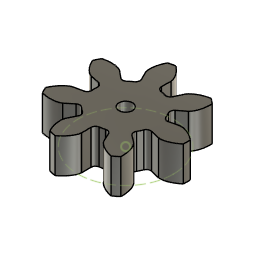
Motor Gear v04 (Autodesk Fusion 360 design; units mm, degrees)
description: Spur Gear; Module: 5.0; Num Teeth: 7; Pressure Angle: 20.0; Backlash: 0.00 mm
Autodesk Fusion 360 part; units mm, degrees
sketch "Sketch1" plane through (0, 0, 0) normal (0, 0, 1) x (1, 0, 0) in component "Spur Gear (7 teeth)"
  circle A0 centre (0, 0) radius 11.4492
  circle A1 centre (0, 0) radius 2.5
extrude "Extrude1" add sketch "Sketch1" along normal blind 12.7 in component "Spur Gear (7 teeth)"
sketch "Sketch2" plane through (0, 0, 0) normal (0, 0, 1) x (1, 0, 0) in component "Spur Gear (7 teeth)"
  spline S0 degree 5 poles (15.976, -3.8978) (15.9941, -3.9022) (16.0303, -3.9103) (16.085, -3.9201) (16.1585, -3.9291) (16.2513, -3.9345) (16.3447, -3.936) (16.4386, -3.9351) (16.5326, -3.9328) (16.6268, -3.9296) (16.7211, -3.9253) (16.8156, -3.9196) (16.9102, -3.912) (17.0051, -3.9022) (17.1001, -3.8904) (17.1953, -3.8767) (17.2906, -3.8614) (17.386, -3.8448) (17.4814, -3.827) (17.5768, -3.808) (17.6722, -3.7879) (17.7676, -3.7664) (17.8631, -3.7436) (17.9586, -3.7194) (18.054, -3.694) (18.1494, -3.6672) (18.2448, -3.6393) (18.3402, -3.6102) (18.4355, -3.58) (18.5307, -3.5487) (18.6259, -3.5163) (18.7209, -3.4828) (18.8159, -3.4482) (18.9108, -3.4124) (19.0056, -3.3756) (19.1003, -3.3378) (19.1948, -3.2988) (19.2893, -3.2589) (19.3835, -3.2179) (19.4777, -3.1759) (19.5717, -3.133) (19.6655, -3.089) (19.7592, -3.044) (19.8527, -2.9981) (19.946, -2.9512) (20.0392, -2.9033) (20.1321, -2.8545) (20.2249, -2.8047) (20.3175, -2.7541) (20.4098, -2.7024) (20.502, -2.6499) (20.5939, -2.5964) (20.6856, -2.5421) (20.7771, -2.4868) (20.8683, -2.4307) (20.9593, -2.3737) (21.05, -2.3157) (21.1405, -2.257) (21.2307, -2.1973) (21.3207, -2.1368) (21.4104, -2.0754) (21.4998, -2.0132) (21.589, -1.9502) (21.6778, -1.8863) (21.7664, -1.8215) (21.8547, -1.756) (21.9427, -1.6896) (22.0303, -1.6224) (22.1177, -1.5544) (22.2047, -1.4857) (22.2915, -1.4161) (22.3606, -1.3598) (22.4123, -1.3172) (22.4467, -1.2886) (22.4639, -1.2743) knots 0 0 0 0 0 0 0.01428571 0.02857143 0.04285714 0.05714286 0.07142857 0.08571429 0.1 0.11428571 0.12857143 0.14285714 0.15714286 0.17142857 0.18571429 0.2 0.21428571 0.22857143 0.24285714 0.25714286 0.27142857 0.28571429 0.3 0.31428571 0.32857143 0.34285714 0.35714286 0.37142857 0.38571429 0.4 0.41428571 0.42857143 0.44285714 0.45714286 0.47142857 0.48571429 0.5 0.51428571 0.52857143 0.54285714 0.55714286 0.57142857 0.58571429 0.6 0.61428571 0.62857143 0.64285714 0.65714286 0.67142857 0.68571429 0.7 0.71428571 0.72857143 0.74285714 0.75714286 0.77142857 0.78571429 0.8 0.81428571 0.82857143 0.84285714 0.85714286 0.87142857 0.88571429 0.9 0.91428571 0.92857143 0.94285714 0.95714286 0.97142857 0.98571429 1 1 1 1 1 1
  spline S1 degree 5 poles (15.976, 3.8978) (15.9941, 3.9022) (16.0303, 3.9103) (16.085, 3.9201) (16.1585, 3.9291) (16.2513, 3.9345) (16.3447, 3.936) (16.4386, 3.9351) (16.5326, 3.9328) (16.6268, 3.9296) (16.7211, 3.9253) (16.8156, 3.9196) (16.9102, 3.912) (17.0051, 3.9022) (17.1001, 3.8904) (17.1953, 3.8767) (17.2906, 3.8614) (17.386, 3.8448) (17.4814, 3.827) (17.5768, 3.808) (17.6722, 3.7879) (17.7676, 3.7664) (17.8631, 3.7436) (17.9586, 3.7194) (18.054, 3.694) (18.1494, 3.6672) (18.2448, 3.6393) (18.3402, 3.6102) (18.4355, 3.58) (18.5307, 3.5487) (18.6259, 3.5163) (18.7209, 3.4828) (18.8159, 3.4482) (18.9108, 3.4124) (19.0056, 3.3756) (19.1003, 3.3378) (19.1948, 3.2988) (19.2893, 3.2589) (19.3835, 3.2179) (19.4777, 3.1759) (19.5717, 3.133) (19.6655, 3.089) (19.7592, 3.044) (19.8527, 2.9981) (19.946, 2.9512) (20.0392, 2.9033) (20.1321, 2.8545) (20.2249, 2.8047) (20.3175, 2.7541) (20.4098, 2.7024) (20.502, 2.6499) (20.5939, 2.5964) (20.6856, 2.5421) (20.7771, 2.4868) (20.8683, 2.4307) (20.9593, 2.3737) (21.05, 2.3157) (21.1405, 2.257) (21.2307, 2.1973) (21.3207, 2.1368) (21.4104, 2.0754) (21.4998, 2.0132) (21.589, 1.9502) (21.6778, 1.8863) (21.7664, 1.8215) (21.8547, 1.756) (21.9427, 1.6896) (22.0303, 1.6224) (22.1177, 1.5544) (22.2047, 1.4857) (22.2915, 1.4161) (22.3606, 1.3598) (22.4123, 1.3172) (22.4467, 1.2886) (22.4639, 1.2743) knots 0 0 0 0 0 0 0.01428571 0.02857143 0.04285714 0.05714286 0.07142857 0.08571429 0.1 0.11428571 0.12857143 0.14285714 0.15714286 0.17142857 0.18571429 0.2 0.21428571 0.22857143 0.24285714 0.25714286 0.27142857 0.28571429 0.3 0.31428571 0.32857143 0.34285714 0.35714286 0.37142857 0.38571429 0.4 0.41428571 0.42857143 0.44285714 0.45714286 0.47142857 0.48571429 0.5 0.51428571 0.52857143 0.54285714 0.55714286 0.57142857 0.58571429 0.6 0.61428571 0.62857143 0.64285714 0.65714286 0.67142857 0.68571429 0.7 0.71428571 0.72857143 0.74285714 0.75714286 0.77142857 0.78571429 0.8 0.81428571 0.82857143 0.84285714 0.85714286 0.87142857 0.88571429 0.9 0.91428571 0.92857143 0.94285714 0.95714286 0.97142857 0.98571429 1 1 1 1 1 1
  arc A0 (22.4639, -1.2743) -> (22.4639, 1.2743) centre (0, 0) ccw
  line L0 (11.1132, -2.7138) -> (15.976, -3.8978)
  line L1 (11.1132, 2.7138) -> (15.976, 3.8978)
  line L2 (11.1132, -2.7138) -> (11.1132, 2.7138)
  point P0 (16.412, -3.9351)
  point P1 (16.861, -3.9157)
  point P2 (17.318, -3.8565)
  point P3 (17.7809, -3.763)
  point P4 (18.2481, -3.638)
  point P5 (18.7184, -3.4834)
  point P6 (19.1906, -3.3003)
  point P7 (19.6636, -3.0896)
  point P8 (20.1364, -2.852)
  point P9 (20.608, -2.5879)
  point P10 (21.0776, -2.2977)
  point P11 (21.544, -1.9818)
  point P12 (22.0064, -1.6406)
  point P13 (16.412, 3.9351)
  point P14 (16.861, 3.9157)
  point P15 (17.318, 3.8565)
  point P16 (17.7809, 3.763)
  point P17 (18.2481, 3.638)
  point P18 (18.7184, 3.4834)
  point P19 (19.1906, 3.3003)
  point P20 (19.6636, 3.0896)
  point P21 (20.1364, 2.852)
  point P22 (20.608, 2.5879)
  point P23 (21.0776, 2.2977)
  point P24 (21.544, 1.9818)
  point P25 (22.0064, 1.6406)
extrude "Extrude2" add sketch "Sketch2" along normal blind 12.7 in component "Spur Gear (7 teeth)"
fillet "Fillet1" radius 1.5875 2 edges at (11.1224, -2.716, 6.35) (11.1224, 2.716, 6.35) in component "Spur Gear (7 teeth)"
pattern_circular "C-Pattern1" count 7 over 360 about axis through (0, 0, 0) along (0, 0, 1) of "Extrude2", "Fillet1" in component "Spur Gear (7 teeth)"
sketch "Sketch3" plane through (0, 0, 0) normal (0, 0, 1) x (1, 0, 0) in component "Spur Gear (7 teeth)"
  circle A0 centre (0, 0) radius 17.5 construction
component "Spur Gear (7 teeth)" placed x (1, 0, 0) y (0, 1, 0) z (0, 0, 1) at (0, 0, 0)
